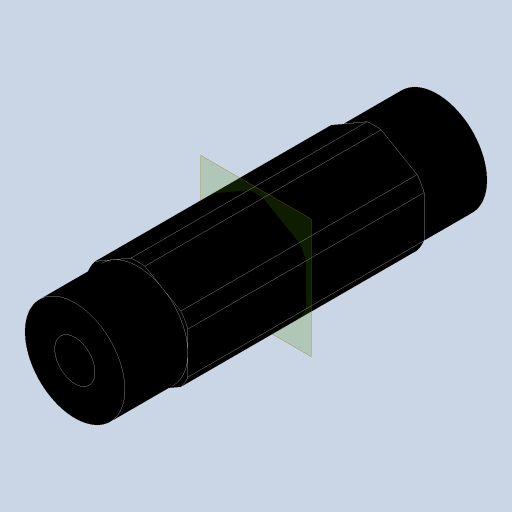
# Autodesk Inventor part: GP5-029
Saved by Autodesk Inventor 2023.4 (Build 274418000, 418)
## iProperties
Created: 2025-02-07
Part Number: GP5-029
Material: Aluminum 6061
Document SubType Name: Modeling
Designer: mavericks
Mass: 8.50758 g
Surface Area: 25.7449 cm^2
Volume: 3.15096 cm^3
Density: 2.7 g/cm^3
Appearance: Anodized - Black
RuleStatus: InUse
AfterDocNew0: SHOW
AfterDocOpen0: SHOW
AfterDocOpen1: size
AfterDocOpen2: thunder
BeforeDocSave0: size
BeforeDocSave1: thunder
AfterFeatureSuppressionChange0: thunder
AfterFeatureSuppressionChange1: size
PartBodyChanged0: thunder
PartBodyChanged1: size
AfterMaterialChange0: thunder
AfterMaterialChange1: size
Author: mavericks
Autodesk Inventor part; units mm, degrees
ref_plane "YZ Plane" through (0, 0, 0) normal (1, 0, 0) x (0, 1, 0)
ref_plane "XZ Plane" through (0, 0, 0) normal (0, 1, 0) x (-1, 0, 0)
ref_plane "XY Plane" through (0, 0, 0) normal (0, 0, 1) x (1, 0, 0)
sketch "Sketch1" plane through (0, 0, 0) normal (0, 0, 1) x (1, 0, 0)
  line L0 (-6.35, -3.6662) -> (-6.35, 3.6662)
  line L1 (-6.35, 3.6662) -> (0, 7.3323)
  line L2 (0, 7.3323) -> (6.35, 3.6662)
  line L3 (6.35, 3.6662) -> (6.35, -3.6662)
  line L4 (6.35, -3.6662) -> (0, -7.3323)
  line L5 (0, -7.3323) -> (-6.35, -3.6662)
  point P0 (0, 0)
  point P1 (0, 0)
  dimension "Size" = 12.7
  constraints: 12 end point, 1 coincident, 1 vertical alignment, 13 other
  measures "Size" distance between parallel lines of L3 L0
extrude "Extrusion1" add sketch "Sketch1" along normal mid plane 45.9994
sketch "Sketch3" plane through (0, 0, 22.9997) normal (0, 0, 1) x (1, 0, 0)
  line L0 (-6.35, 3.6662) -> (0, 7.3323) construction
  line L1 (0, 7.3323) -> (6.35, 3.6662) construction
  line L2 (6.35, 3.6662) -> (6.35, -3.6662) construction
  line L3 (6.35, -3.6662) -> (0, -7.3323) construction
  line L4 (0, -7.3323) -> (-6.35, -3.6662) construction
  line L5 (-6.35, -3.6662) -> (-6.35, 3.6662) construction
  point P0 (0, 0)
hole "Hole1" at (0, 0, 22.9997) direction (0, 0, -1) diameter 5.1054 end through all
sketch "Sketch4" plane through (0, 0, 22.9997) normal (0, 0, 1) x (1, 0, 0)
  circle A0 centre (0, 0) radius 2.5527 construction
  line L0 (-6.35, 3.6662) -> (0, 7.3323) construction
  line L1 (0, 7.3323) -> (6.35, 3.6662) construction
  line L2 (6.35, 3.6662) -> (6.35, -3.6662) construction
  line L3 (6.35, -3.6662) -> (0, -7.3323) construction
  line L4 (0, -7.3323) -> (-6.35, -3.6662) construction
  line L5 (-6.35, -3.6662) -> (-6.35, 3.6662) construction
  circle A1 centre (0, 0) radius 6.8771
  circle A2 centre (0, 0) radius 8.89
  dimension "thunder" = 13.7541
  dimension "d16" = 17.78
  constraints: 2 centre point, 2 coincident
  measures "thunder" diameter of A1
  measures "d16" diameter of A2
extrude "Extrusion3" cut sketch "Sketch4" against normal through all
sketch "Sketch5" plane through (0, 0, 22.9997) normal (0, 0, 1) x (1, 0, 0)
  circle A0 centre (0, 0) radius 6.35
  arc A1 (5.4616, -4.1791) -> (6.35, -2.6403) centre (0, 0) ccw projected
  line L0 (6.35, -2.6403) -> (6.35, 2.6403) projected
  arc A2 (6.35, 2.6403) -> (5.4616, 4.1791) centre (0, 0) ccw projected
  line L1 (5.4616, 4.1791) -> (0.8884, 6.8194) projected
  arc A3 (0.8884, 6.8194) -> (-0.8884, 6.8194) centre (0, 0) ccw projected
  line L2 (-0.8884, 6.8194) -> (-5.4616, 4.1791) projected
  arc A4 (-5.4616, 4.1791) -> (-6.35, 2.6403) centre (0, 0) ccw projected
  line L3 (-6.35, 2.6403) -> (-6.35, -2.6403) projected
  arc A5 (-6.35, -2.6403) -> (-5.4616, -4.1791) centre (0, 0) ccw projected
  line L4 (-5.4616, -4.1791) -> (-0.8884, -6.8194) projected
  arc A6 (-0.8884, -6.8194) -> (0.8884, -6.8194) centre (0, 0) ccw projected
  line L5 (0.8884, -6.8194) -> (5.4616, -4.1791) projected
  circle A7 centre (0, 0) radius 2.5527 projected
  point P0 (3.175, -5.4993)
  point P1 (-3.175, -5.4993)
  point P2 (-6.35, 0)
  point P3 (-3.175, 5.4993)
  point P4 (3.175, 5.4993)
  point P5 (6.35, 0)
  dimension "d19" = 12.7
  constraints: 1 centre point, 1 coincident
  measures "d19" diameter of A0
extrude "Extrusion4" cut sketch "Sketch5" against normal blind 8.001 contours L0 A1 L5 A0 | A0 L1 A2 L0 | A0 L2 A3 L1 | L5 A6 L4 A0 | A0 L3 A4 L2 | L4 A5 L3 A0
mirror "Mirror2" about plane through (0, 0, 0) normal (0, 0, 1) of "Extrusion4"
ref_plane "Work Plane1" through (0, 0, 0) normal (0, 0, 1) x (1, 0, 0)
equation "\"bearing\" = 25.4"
body "Solid1"
